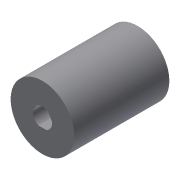
# Autodesk Inventor part: OPENTRONS_Autofocus_clutch_Nema
Saved by Autodesk Inventor 2019.4 (Build 234330000, 330)
## iProperties
Created: 2021-01-06
Part Number: OPENTRONS_Autofocus_clutch_Nema
Material: Generic
Document SubType Name: Modeling
Designer: diederichbenedict
Density: 1 g/cm^3
Appearance: Default
Author: diederichbenedict
Autodesk Inventor part; units mm, degrees
ref_plane "YZ Plane" through (0, 0, 0) normal (1, 0, 0) x (0, 1, 0)
ref_plane "XZ Plane" through (0, 0, 0) normal (0, 1, 0) x (-1, 0, 0)
ref_plane "XY Plane" through (0, 0, 0) normal (0, 0, 1) x (1, 0, 0)
sketch "Sketch1" plane through (0, 0, 0) normal (0, 0, 1) x (1, 0, 0)
  circle A0 centre (0, 0) radius 2.5 projected
  circle A1 centre (0, 0) radius 2.6
  line L0 (-1.3981, 2.1921) -> (1.3981, 2.1921)
  circle A2 centre (0, 0) radius 5
  dimension "d0" = 0.1
  dimension "d1" = 10
  constraints: 2 centre point, 2 end point, 2 point on circle, 1 coincident, 1 horizontal
  measures "d0" radial gap between concentric circles of A0 A1
  measures "d1" diameter of A2
extrude "Extrusion1" add sketch "Sketch1" against normal blind 10
sketch "Sketch2" plane through (0, 0, 0) normal (0, 0, 1) x (1, 0, 0)
  circle A0 centre (0, 0) radius 1.4 construction
  line L0 (0.6514, -1.4) -> (-0.6514, -1.4)
  line L1 (1.5381, 0.1359) -> (0.8867, 1.2641)
  line L2 (-0.8867, 1.2641) -> (-1.5381, 0.1359)
  arc A1 (0.6514, -1.4) -> (1.5381, 0.1359) centre (0, 0) ccw
  arc A2 (-1.5381, 0.1359) -> (-0.6514, -1.4) centre (0, 0) ccw
  arc A3 (0.8867, 1.2641) -> (-0.8867, 1.2641) centre (0, 0) ccw
  circle A4 centre (0, 0) radius 5 projected
  dimension "d4" = 2.8
  dimension "d9" = 60
  dimension "d10" = 60
  constraints: 6 end point, 6 point on circle, 4 centre point, 3 tangent, 1 coincident, 1 horizontal
  measures "d4" diameter of A0
  measures "d9" angle of L1 L0
  measures "d10" angle of L2 L0
extrude "Extrusion2" add sketch "Sketch2" along normal blind 5
sketch "Sketch3" plane through (0, 0, -10) normal (0, 0, -1) x (-1, 0, 0)
  line L0 (-2.1363, -1.482) -> (-2.1363, 1.482)
  circle A0 centre (0, 0) radius 2.6 projected
  constraints: 2 end point, 2 point on circle, 1 vertical
extrude "Extrusion3" add sketch "Sketch3" against normal up to surface (10 mm away) contours A0 L0 picked at (-2.2341, 0.3085)
body "Solid1"
